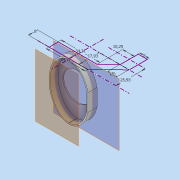
# Autodesk Inventor part: lw_4_крепление
Saved by Autodesk Inventor 2019 (Build 230136000, 136)
## iProperties
Created: 2021-03-07
Part Number: lw_4_крепление
Material: Типовые
Document SubType Name: Modeling
Designer: Kurbatova
Density: 1 g/cm^3
Appearance: По умолчанию
Author: Kurbatova
Autodesk Inventor part; units mm, degrees
ref_plane "YZ Plane" through (0, 0, 0) normal (1, 0, 0) x (0, 1, 0)
ref_plane "XZ Plane" through (0, 0, 0) normal (0, 1, 0) x (-1, 0, 0)
sketch "Эскиз1" plane through (0, 0, 0) normal (0, 1, 0) x (-1, 0, 0)
  line L0 (21.012709, -18.110161) -> (-13.297291, -18.110161)
  line L1 (21.012709, -18.110161) -> (21.012709, -10.110161)
  line L2 (21.012709, -10.110161) -> (-13.297291, -10.110161)
  line L3 (20.45098, -28.040161) -> (-43.624294, -28.040161)
  line L4 (-23.547291, -28.040161) -> (-23.547291, -44.040161)
  line L5 (-23.547291, -44.040161) -> (-31.547291, -44.040161)
  line L6 (-31.547291, -44.040161) -> (-31.547291, -28.040161)
  line L7 (-31.547291, -28.040161) -> (-13.297291, -10.110161)
  line L8 (-23.547291, -28.040161) -> (-13.297291, -18.110161)
  line L9 (-5.229325, -36.040161) -> (-38.076533, -36.040161)
  line L10 (31.384679, -10.110161) -> (-49.584403, -10.110161)
  line L11 (3.155484, -40.25251) -> (3.155484, 5.516657)
  point P0 (0, 0)
  point P1 (-23.547291, -36.040161)
  dimension "d0" = 34.31
  dimension "d2" = 8
  dimension "d3" = 34.31
  dimension "d5" = 8
  dimension "d7" = 17.93
  dimension "d8" = 25.93
  dimension "d9" = 10.25
  dimension "d10" = 8
  constraints: 24 end point, 4 perpendicular, 4 point on line, 3 horizontal, 3 vertical, 1 midpoint
  measures "d0" distance of L0.start L0.end
  measures "d2" distance of L0.start L1.end
  measures "d3" distance of L1.end L2.end
  measures "d5" distance of L4.end L5.end
  measures "d7" vertical distance of L6.end L2.end
  measures "d8" distance between parallel lines of L10 L9
  measures "d9" distance from line of L0.end L4
  measures "d10" distance of L6.end L4.start
extrude "Выдавливание1" add sketch "Эскиз1" against normal blind 49.99 contours L0 L11 L2 L1 | L0 L8 L3 L7 L2 L11 | L4 L9 L6 L3 | L4 L5 L6 L9
ref_plane "РабПлоскость4" through (13.297291, 0, -14.110161) normal (0, 0, -1) x (-1, 0, 0)
sketch "Эскиз7" plane through (13.297291, 0, -18.110161) normal (0, 0, -1) x (-1, 0, 0)
  line L0 (0, 0) -> (0, -49.99)
  line L1 (17.155, -59.591206) -> (17.155, 20.47264)
  line L2 (47.826802, -24.995) -> (-14.329584, -24.995)
  line L3 (0, 0) -> (34.31, 0)
  line L4 (34.31, -49.99) -> (0, -49.99)
  ellipse E0 centre (16.748609, -24.995) end of major axis (34.307254, -25.213135) minor radius 24.998492 (0, -32.725087) -> (0, -17.692011) ccw
  line L5 (34.31, 0) -> (34.31, -49.99)
  circle A0 centre (16.748609, -24.995) radius 12.5
  ellipse E1 centre (16.748609, -24.995) end of major axis (34.307254, -25.213135) minor radius 24.998492 (0, -32.725087) -> (16.342218, -49.99) ccw
  point P0 (0, -24.995)
  point P1 (17.155, 0)
  dimension "d29" = 17.56
  dimension "d31" = 25
  constraints: 5 point on line, 4 end point, 3 midpoint, 2 vertical, 1 centre point, 1 coincident, 1 horizontal, 9 other
  measures "d31" diameter of A0
extrude "Выдавливание2" cut sketch "Эскиз7" against normal blind 45 contours E0 L3 L1 A0 L2 L0 | L2 A0 L1 E0 L4 L0 | E0 L2 A0 L1 | A0 L2 E0 L1 keep common part
shell "Оболочка1" thickness 1 removed faces 2 at (-15.789446, -27.000141, -12.776828) at (11.881088, -25.137366, -10.110161)
